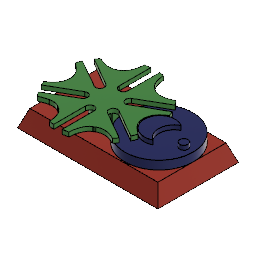
crank+wheel (Autodesk Fusion 360 design; units mm, degrees)
Autodesk Fusion 360 part; units mm, degrees
note: some values were not read from the file. Chosen so that the rebuilt part matches the saved one: the sign of a taper. Set by a fixed rule: which sketch regions a step uses.
sketch "Base" plane through (0, 0, 0) normal (0, 0, 1) x (1, 0, 0)
  line L0 (90, -40) -> (-60, -40)
  line L1 (-60, 40) -> (90, 40)
  line L2 (90, 40) -> (90, -40)
  line L3 (-60, 40) -> (-60, -40)
  constraint horizontal L0
  constraint parallel L0 L1
  constraint perpendicular L0 L3
extrude "Extrude1" add sketch "Base" along normal blind 20 contours L0 L1 L2 L3 picked at (40, -13.333333) makes body 1
draft "Draft1" angle -20 neutral plane through (0, 0, 20) pull (0, 0, -1) 1 faces at (90, 13.333333, 6.666667) on bodies 1
draft "Draft2" angle -20 neutral plane through (0, 0, 20) pull (0, 0, -1) 1 faces at (42.426468, -40, 6.666667) on bodies 1
draft "Draft4" angle -20 neutral plane through (0, 0, 20) pull (0, 0, -1) 1 faces at (42.426468, 40, 6.666667) on bodies 1
sketch "Support" plane through (0, 0, 20) normal (0, 0, 1) x (-1, 0, 0)
  line L0 (-90, -40) -> (60, -40)
  line L1 (60, 40) -> (-90, 40)
  line L2 (-90, 40) -> (-90, -40)
  circle A0 centre (-51, 0) radius 5
  line L3 (60, -40) -> (60, 40)
  dimension "d19" = 10
  dimension "d22" = 39
  measures "d19" diameter of A0
  measures "d22" distance of L2 A0.centre
sketch "Crank" plane through (0, 0, 20) normal (0, 0, 1) x (-1, 0, 0)
  line L0 (-90, -40) -> (60, -40)
  line L1 (60, 40) -> (-90, 40)
  line L2 (-90, 40) -> (-90, -40)
  circle A0 centre (-50, 0) radius 40
  circle A1 centre (-50, 0) radius 5
  line L3 (60, -40) -> (60, 40)
  dimension "d24" = 80
  dimension "d25" = 10
  constraint concentric A0 A1
  measures "d24" diameter of A0
  measures "d25" diameter of A1
extrude "Extrude5" add sketch "Crank" along normal blind 10 separate body contours A0 picked at (-47.977919, -28.192959) makes body 2
move_body "Move1" bodies 2 to x (0.81915204, 0.57357644, 0) y (-0.57357644, 0.81915204, 0) z (0, 0, 1) at (9.093093, -27.45285, 0)
sketch "Wheel" plane through (0, 0, 30) normal (0, 0, 1) x (-1, 0, 0)
  circle A0 centre (-50.050695, -1.225972) radius 40
  circle A1 centre (10, 0) radius 15
  line L0 (4.65827, 19.962743) -> (4.65827, 57.25134)
  line L1 (14.65827, 57.310998) -> (14.65827, 19.962743)
  arc A2 (4.65827, 19.962743) -> (14.65827, 19.962743) centre (9.65827, 19.962743) ccw
  line L2 (-9.959108, 5.355298) -> (-42.25198, 23.999596)
  arc A3 (-9.959108, 5.355298) -> (-4.959108, 14.015552) centre (-7.459108, 9.685425) ccw
  line L3 (-41.868798, -24.816885) -> (-7.188355, -5.277822)
  arc A4 (-4.617378, -14.607445) -> (-7.188355, -5.277822) centre (-7.117378, -10.277318) ccw
  line L4 (5.34173, -57.310998) -> (5.34173, -19.962743)
  line L5 (15.34173, -19.962743) -> (15.34173, -57.25134)
  arc A5 (15.34173, -19.962743) -> (5.34173, -19.962743) centre (10.34173, -19.962743) ccw
  line L6 (57.303653, -32.689684) -> (24.959108, -14.015552)
  line L7 (29.959108, -5.355298) -> (62.251987, -23.999601)
  arc A6 (29.959108, -5.355298) -> (24.959108, -14.015552) centre (27.459108, -9.685425) ccw
  line L8 (61.961916, 24.621319) -> (29.617378, 5.947191)
  line L9 (24.617378, 14.607445) -> (56.91025, 33.251744)
  arc A7 (24.617378, 14.607445) -> (29.617378, 5.947191) centre (27.117378, 10.277318) ccw
  arc A8 (-28.748606, 16.20342) -> (-28.323248, -17.185283) centre (10, 0) ccw
  line L10 (-36.348989, 10.447213) -> (-36.348989, 10.647333)
  spline S0 degree 5 poles (-31.998652, -0.344178) (-31.992978, -0.42935) (-31.981962, -0.599616) (-31.966433, -0.854778) (-31.947856, -1.194487) (-31.929918, -1.617863) (-31.922458, -1.95492) (-31.922684, -2.206325) (-31.925837, -2.373212) (-31.928165, -2.456477) knots 0 0 0 0 0 0 0.2 0.4 0.6 0.8 1 1 1 1 1 1
  line L11 (-31.922228, -2.244113) -> (-31.934101, -2.668841)
  arc A9 (42.395294, 34.815724) -> (42.395392, 34.815743) centre (39.007339, 52.494009) ccw
  spline S1 degree 5 poles (42.395294, 34.815724) (42.395299, 34.815725) (42.395309, 34.815727) (42.395322, 34.815729) (42.395334, 34.815732) (42.395343, 34.815733) (42.395349, 34.815735) (42.395354, 34.815736) (42.395363, 34.815737) (42.395378, 34.815741) (42.395405, 34.815746) (42.395438, 34.815752) (42.395471, 34.815758) (42.395497, 34.815763) (42.395511, 34.815766) knots 0 0 0 0 0 0 0.1 0.2 0.3 0.4 0.5 0.6 0.7 0.8 0.9 1 1 1 1 1 1
  line L12 (42.395245, 34.815715) -> (42.395343, 34.815733)
  line L13 (42.395462, 34.815756) -> (42.39556, 34.815775)
  arc A10 (-23.406876, -25.455567) -> (5.721267, -41.781547) centre (10, 0) ccw
  arc A11 (15.34173, -41.658987) -> (44.044515, -24.596265) centre (10, 0) ccw
  arc A12 (48.748606, -16.20342) -> (48.323248, 17.185282) centre (10, 0) ccw
  arc A13 (43.406876, 25.455567) -> (14.278733, 41.781547) centre (10, 0) ccw
  arc A14 (4.65827, 41.658987) -> (-24.044515, 24.596265) centre (10, 0) ccw
  arc A15 (64.101973, 19.473739) -> (61.961916, 24.621319) centre (10, 0) ccw
  spline S2 degree 5 poles (51.998652, 0.344178) (51.948747, 1.004913) (51.912096, 2.317577) (52.046589, 4.260157) (52.611126, 6.796556) (53.995667, 9.872405) (56.099598, 12.847954) (58.582809, 15.357591) (60.893976, 17.237438) (62.700289, 18.533897) (63.801488, 19.274887) (64.101973, 19.473739) knots 0 0 0 0 0 0 0.1 0.2 0.3 0.4 0.5 0.6 0.63682387 0.63682387 0.63682387 0.63682387 0.63682387 0.63682387
  line L14 (61.633649, 17.840284) -> (66.570298, 21.107194)
  spline S3 degree 5 poles (30.70126, 36.543989) (31.182546, 36.238047) (32.176219, 35.680024) (33.760026, 35.004552) (36.061496, 34.432479) (39.27183, 34.294915) (42.833861, 34.766393) (46.268412, 35.720002) (49.109414, 36.785143) (51.197349, 37.685575) (52.436845, 38.256139) (52.782265, 38.417805) knots 0 0 0 0 0 0 0.1 0.2 0.3 0.4 0.5 0.6 0.63831038 0.63831038 0.63831038 0.63831038 0.63831038 0.63831038
  line L15 (50.364178, 37.286076) -> (55.200353, 39.549535)
  spline S4 degree 5 poles (30.70126, 36.543989) (30.104094, 36.831137) (28.948967, 37.455728) (27.33389, 38.543493) (25.419573, 40.300595) (23.44808, 43.037567) (21.923145, 46.347399) (20.991341, 49.752743) (20.518928, 52.694195) (20.299319, 54.906738) (20.208202, 56.230899) (20.186234, 56.590553) knots 0 0 0 0 0 0 0.1 0.2 0.3 0.4 0.5 0.6 0.63682387 0.63682387 0.63682387 0.63682387 0.63682387 0.63682387
  line L16 (20.364483, 53.672257) -> (20.007985, 59.508849)
  arc A16 (56.91025, 33.251744) -> (52.782265, 38.417805) centre (10, 0) ccw
  arc A17 (20.186234, 56.590553) -> (14.65827, 57.310998) centre (10, 0) ccw
  spline S5 degree 5 poles (-11.297393, 36.199811) (-10.791797, 36.463646) (-9.811697, 37.045181) (-8.434818, 38.079062) (-6.788654, 39.786157) (-5.064352, 42.497606) (-3.691649, 45.818154) (-2.800223, 49.269367) (-2.302161, 52.262318) (-2.037991, 54.520739) (-1.912366, 55.879456) (-1.879663, 56.259431) knots 0 0 0 0 0 0 0.1 0.2 0.3 0.4 0.5 0.6 0.63831039 0.63831039 0.63831039 0.63831039 0.63831039 0.63831039
  line L17 (-2.124356, 53.416371) -> (-1.634969, 59.102492)
  arc A18 (4.65827, 57.25134) -> (-1.879663, 56.259431) centre (10, 0) ccw
  spline S6 degree 5 poles (-11.297393, 36.199811) (-11.844654, 35.826225) (-12.963128, 35.138151) (-14.712699, 34.283336) (-17.191553, 33.504039) (-20.547586, 33.165163) (-24.176453, 33.499446) (-27.591469, 34.395152) (-30.375047, 35.456757) (-32.40097, 36.372841) (-33.593286, 36.956011) (-33.915739, 37.116814) knots 0 0 0 0 0 0 0.1 0.2 0.3 0.4 0.5 0.6 0.63682387 0.63682387 0.63682387 0.63682387 0.63682387 0.63682387
  line L18 (-31.532038, 35.928099) -> (-36.29944, 38.305529)
  line L19 (-37.303645, 32.689679) -> (-4.959108, 14.015552)
  arc A19 (-33.915739, 37.116814) -> (-37.303645, 32.68968) centre (10, 0) ccw
  spline S7 degree 5 poles (-31.998652, -0.344178) (-31.974342, 0.225599) (-31.987917, 1.365158) (-32.194845, 3.07451) (-32.850149, 5.353678) (-34.336183, 8.202691) (-36.52551, 11.051761) (-39.068635, 13.549365) (-41.411576, 15.477175) (-43.23534, 16.835164) (-44.349211, 17.623316) (-44.661928, 17.841626) knots 0 0 0 0 0 0 0.1 0.2 0.3 0.4 0.5 0.6 0.63831039 0.63831039 0.63831039 0.63831039 0.63831039 0.63831039
  line L20 (-42.270807, 16.172369) -> (-47.053049, 19.510883)
  arc A20 (-42.25198, 23.999596) -> (-44.661928, 17.841626) centre (10, 0) ccw
  spline S8 degree 5 poles (-31.998652, -0.344178) (-31.948747, -1.004913) (-31.912096, -2.317577) (-32.046589, -4.260157) (-32.611126, -6.796556) (-33.995667, -9.872405) (-36.099598, -12.847954) (-38.582809, -15.357591) (-40.893976, -17.237438) (-42.70029, -18.533897) (-43.801488, -19.274888) (-44.101974, -19.473739) knots 0 0 0 0 0 0 0.1 0.2 0.3 0.4 0.5 0.6 0.63682388 0.63682388 0.63682388 0.63682388 0.63682388 0.63682388
  line L21 (-41.633649, -17.840284) -> (-46.570298, -21.107194)
  line L22 (-4.617378, -14.607445) -> (-36.91025, -33.251744)
  arc A21 (-44.101974, -19.473739) -> (-41.868799, -24.816885) centre (10, 0) ccw
  spline S9 degree 5 poles (-10.70126, -36.543989) (-11.182546, -36.238047) (-12.17622, -35.680024) (-13.760026, -35.004552) (-16.061496, -34.432479) (-19.27183, -34.294915) (-22.833861, -34.766393) (-26.268412, -35.720002) (-29.109414, -36.785143) (-31.197349, -37.685575) (-32.436845, -38.25614) (-32.782266, -38.417805) knots 0 0 0 0 0 0 0.1 0.2 0.3 0.4 0.5 0.6 0.63831039 0.63831039 0.63831039 0.63831039 0.63831039 0.63831039
  line L23 (-30.364178, -37.286076) -> (-35.200353, -39.549535)
  arc A22 (-36.91025, -33.251744) -> (-32.782266, -38.417805) centre (10, 0) ccw
  spline S10 degree 5 poles (-10.70126, -36.543989) (-10.104094, -36.831137) (-8.948967, -37.455728) (-7.33389, -38.543493) (-5.419573, -40.300595) (-3.44808, -43.037567) (-1.923145, -46.347399) (-0.991341, -49.752743) (-0.518928, -52.694195) (-0.299319, -54.906738) (-0.208202, -56.230899) (-0.186234, -56.590553) knots 0 0 0 0 0 0 0.1 0.2 0.3 0.4 0.5 0.6 0.63682387 0.63682387 0.63682387 0.63682387 0.63682387 0.63682387
  line L24 (-0.364483, -53.672257) -> (-0.007986, -59.508849)
  arc A23 (-0.186234, -56.590553) -> (5.34173, -57.310998) centre (10, 0) ccw
  spline S11 degree 5 poles (31.297393, -36.199811) (30.791797, -36.463646) (29.811697, -37.045181) (28.434818, -38.079062) (26.788654, -39.786157) (25.064352, -42.497606) (23.691649, -45.818154) (22.800223, -49.269367) (22.302161, -52.262318) (22.037991, -54.520739) (21.912366, -55.879456) (21.879663, -56.259432) knots 0 0 0 0 0 0 0.1 0.2 0.3 0.4 0.5 0.6 0.63831039 0.63831039 0.63831039 0.63831039 0.63831039 0.63831039
  line L25 (22.124356, -53.416371) -> (21.634969, -59.102492)
  arc A24 (15.34173, -57.25134) -> (21.879663, -56.259431) centre (10, 0) ccw
  spline S12 degree 5 poles (31.297393, -36.199811) (31.844653, -35.826225) (32.963128, -35.138151) (34.712699, -34.283336) (37.191553, -33.504039) (40.547586, -33.165163) (44.176453, -33.499446) (47.59147, -34.395152) (50.37505, -35.456758) (52.400975, -36.372843) (53.593292, -36.956015) (53.915747, -37.116818) knots 0 0 0 0 0 0 0.1 0.2 0.3 0.4 0.5 0.6 0.63682406 0.63682406 0.63682406 0.63682406 0.63682406 0.63682406
  line L26 (51.532045, -35.928102) -> (56.299449, -38.305534)
  arc A25 (53.915747, -37.116818) -> (57.303653, -32.689684) centre (10, 0) ccw
  arc A26 (62.251987, -23.999601) -> (64.661936, -17.841629) centre (10, 0) ccw
  spline S13 degree 5 poles (51.998652, 0.344178) (51.974342, -0.225599) (51.987917, -1.365158) (52.194844, -3.07451) (52.850149, -5.353678) (54.336182, -8.202691) (56.52551, -11.051761) (59.068636, -13.549366) (61.411578, -15.477177) (63.235344, -16.835167) (64.349217, -17.623321) (64.661936, -17.841632) knots 0 0 0 0 0 0 0.1 0.2 0.3 0.4 0.5 0.6 0.63831057 0.63831057 0.63831057 0.63831057 0.63831057 0.63831057
  line L27 (62.270813, -16.172374) -> (67.053058, -19.510889)
  circle A27 centre (10, 0) radius 8.5
  arc A28 (-36.04541, 10.286808) -> (-36.348989, 10.647333) centre (-49.964815, -1.125912) ccw
  arc A29 (-36.349014, -12.899187) -> (-35.640126, -12.025606) centre (-49.964815, -1.125912) ccw
  arc A30 (-31.970459, -1.576656) -> (-32.000063, 0.000007) centre (-49.964815, -1.125912) ccw
  circle A31 centre (-50.050695, -1.225972) radius 5
  point P0 (-36.348989, -12.899158)
  point P1 (42.395355, 34.815736)
  point P2 (-2.003497, -46.588981)
  point P3 (-22.395355, -34.815736)
  point P4 (44.345493, -33.689823)
  point P5 (23.953634, -45.463069)
  point P6 (56.348989, 12.899158)
  point P7 (56.348989, -10.647333)
  point P8 (22.003497, 46.588981)
  point P9 (42.395355, 34.815736)
  point P10 (-24.345493, 33.689823)
  point P11 (-3.953634, 45.463068)
  dimension "d60" = 36
  dimension "d63" = 30
  dimension "d64" = 10
  dimension "d65" = 10
  dimension "d78" = 115
  dimension "d85" = 17
  constraint parallel L0 L1
  constraint vertical L10
  constraint concentric A15 A16
  constraint concentric A16 A17
  constraint concentric A17 A18
  constraint concentric A18 A19
  constraint concentric A19 A20
  constraint concentric A20 A21
  constraint concentric A21 A22
  constraint concentric A22 A23
  constraint concentric A23 A24
  constraint concentric A24 A25
  constraint concentric A25 A26
  constraint concentric A17 A27
  constraint concentric A28 A29
  constraint concentric A29 A30
  measures "d60" diameter of A29
  measures "d63" diameter of A1
  measures "d64" diameter of A2
  measures "d78" diameter of A15
  measures "d85" diameter of A27
sketch "Wheel support" plane through (0, 0, 20) normal (0, 0, 1) x (-1, 0, 0)
  circle A0 centre (10, 0) radius 8.35
  line L0 (-90, 40) -> (-90, -40)
  dimension "d86" = 16.7
  dimension "d109" = 100
  measures "d86" diameter of A0
  measures "d109" distance of A0.centre L0
extrude "Extrude10" add sketch "Wheel support" along normal blind 10 contours A0 picked at (11.887361, -0.51729) bodies 1
extrude "Extrude11" add sketch "Wheel" against normal blind 10 separate body contours A1 A2 A3 A4 A5 A6 A7 picked at (12.871615, 12.482815) makes body 3
extrude "Extrude12" add sketch "Wheel" along normal blind 5 contours A0 L2 L3 A8 S0 L11 S7 S8 A30 | A0 A1 L2 A3 L3 A4 | A0 A14 L19 | A0 A1 L0 A2 A3 A14 S5 S6 L19 | L2 A8 S7 A20 A28 | A0 A1 A4 L4 A5 A10 L22 S9 S10 | A0 A10 L22 | L3 A8 S8 A21 A29 | A0 A14 L19 A19 | A0 A14 S6 A19 | A1 A2 A3 A4 A5 A6 A7 | A0 A10 S9 A22 | A0 A10 L22 A22 | L9 A13 S3 A16 | L0 A14 S5 A18 | A1 L1 A2 L9 A7 A9 A13 S3 S4 | L4 A10 S10 A23 | A1 L5 A5 L6 A6 A11 S11 S12 | A1 L7 A6 L8 A7 A12 S2 S13 | L1 A13 S4 A17 | L5 A11 S11 A24 | L6 A11 S12 A25 | L8 A12 A15 S2 | A9 S3 S4 | L7 A12 A26 S13 | A27 picked at (-24.630972, 3.361792) picked at (-7.648487, 2.202493) picked at (-20.70218, 24.386265) picked at (-3.866077, 23.392702) picked at (-37.478707, 18.548836) picked at (-3.325636, -23.704726) picked at (-19.627621, -24.983172) picked at (-36.235392, -19.05044) picked at (-29.011538, 29.421134) picked at (-23.224268, 30.43015) picked at (12.871615, 12.482815) picked at (-22.249212, -31.758626) picked at (-29.729824, -31.288904) picked at (49.803109, 31.843346) picked at (2.27845, 50.102692) picked at (23.166128, 23.78445) picked at (3.175299, -49.518164) picked at (23.866077, -23.392702) picked at (37.191713, 0.312024) picked at (16.628102, 50.58664) picked at (17.72155, -50.102692) picked at (50.084657, -30.875072) picked at (56.784062, 19.279416) picked at (30.742109, 36.510498) picked at (56.795398, -17.973393) picked at (9.618466, -3.569347) bodies 3
copy_body "Body->Comp7" bodies 2 removing the originals makes body 4 in component "Crank"
copy_body "Body->Comp8" bodies 1 removing the originals makes body 5 in component "Base"
copy_body "Body->Comp9" bodies 3 removing the originals makes body 6 in component "Wheel"
sketch "Crank support" plane through (0, 0, 20) normal (0, 0, 1) x (-1, 0, 0)
  circle A0 centre (10, 0) radius 8.35
  line L0 (-90, -40) -> (60, -40)
  line L1 (60, 40) -> (-90, 40)
  line L2 (-90, 40) -> (-90, -40)
  circle A1 centre (-50.050695, -1.225972) radius 4.85
  line L3 (60, -40) -> (60, 40)
  dimension "d126" = 9.7
  measures "d126" diameter of A1
extrude "Extrude1'" add sketch "Crank support" along normal blind 5 contours A1 picked at (-49.402462, -0.585103) bodies 5 in component "Base"
sketch "Sketch17" plane through (0, 0, 30) normal (0, 0, 1) x (-1, 0, 0)
  circle A0 centre (-50.050695, -1.225972) radius 5
  circle A1 centre (-50.050695, -1.225972) radius 40
  circle A2 centre (-50.050695, -1.225972) radius 5
  constraint concentric A0 A2
extrude "Extrude1''" add sketch "Sketch17" against normal blind 5 contours A0 A2 picked at (-51.336753, -0.518986) bodies 4 in component "Crank"
sketch "Sketch18" plane through (0, 0, 30) normal (0, 0, 1) x (-1, 0, 0)
  circle A0 centre (-50.050695, -1.225972) radius 40
  arc A1 (-44.101974, -19.473739) -> (-41.868799, -24.816885) centre (10, 0) ccw
  line L0 (-4.617378, -14.607445) -> (-36.91025, -33.251744)
  line L1 (-41.868799, -24.816885) -> (-7.188355, -5.277822)
  circle A2 centre (-79.359, -1.032064) radius 4.85
  line L2 (-90, 40) -> (-90, -40)
  arc A3 (-60.982195, -16.078845) -> (-59.194607, 15.04678) centre (-69.073595, 0) ccw
  arc A4 (-60.982195, -16.078845) -> (-59.194607, 15.04678) centre (-51.103207, -1.032064) ccw
  dimension "d131" = 36
  dimension "d132" = 57.5
  dimension "d133" = 0.60296
  dimension "d134" = 9.784377
  dimension "d137" = 9.7
  dimension "d138" = 5.791052
  dimension "d139" = 10.641
  measures "d131" diameter of A4
  measures "d132" radius of A1
  measures "d133" angle of L0 L1
  measures "d137" diameter of A2
extrude "Extrude2" add sketch "Sketch18" along normal blind 5 contours A2 | A3 A4 picked at (-79.630466, -2.383273) picked at (-39.13858, -0.823482) bodies 4 in component "Crank"
draft "Draft1'" angle -20 neutral plane through (0, 0, 20) pull (0, 0, -1) 1 faces at (-60, 13.333333, 6.666667) on bodies 5 in component "Base"
component "Crank" placed x (1, 0, 0) y (0, 1, 0) z (0, 0, 1) at (0, 0, 0)
component "Base" placed x (1, 0, 0) y (0, 1, 0) z (0, 0, 1) at (0, 0, 0)
component "Wheel" placed x (1, 0, 0) y (0, 1, 0) z (0, 0, 1) at (0, 0, 0)
named bodies: "Base", "Crank", "Wheel"
